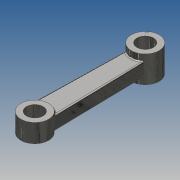
# Autodesk Inventor part: Pleuel_ra8846s
Saved by Autodesk Inventor 2021 (Build 250183000, 183)
## iProperties
Created: 2020-11-17
Part Number: Pleuel_ra8846s
Material: Stahl, hochfest, niedrig legiert
Document SubType Name: Modeling
Designer: Ricardo A
Density: 7.85031 g/cm^3
Appearance: Stahl - poliert
Description: Motor_Teil8_Pleuel
Mass: 3.359 g
Surface Area: 6.12955 cm^2
Volume: 0.427881 cm^3
Author: Sander
Revision Number: Rev00
Autodesk Inventor part; units mm, degrees
ref_plane "YZ-Ebene" through (0, 0, 0) normal (1, 0, 0) x (0, 1, 0)
ref_plane "XZ-Ebene" through (0, 0, 0) normal (0, 1, 0) x (-1, 0, 0)
ref_plane "XY-Ebene" through (0, 0, 0) normal (0, 0, 1) x (1, 0, 0)
sketch "Skizze1" plane through (0, 0, 0) normal (0, 0, 1) x (1, 0, 0)
  line L0 (-3.5, 0) -> (3.5, 0) projected
  line L1 (0, -16.8) -> (0, 16.8) projected
  line L2 (-2, 12) -> (2, 12)
  line L3 (2, 12) -> (2.5, -12)
  line L4 (2.5, -12) -> (-2.5, -12)
  line L5 (-2.5, -12) -> (-2, 12)
  point P0 (0, 0)
  dimension "d0" = 4
  dimension "d1" = 24
  dimension "d2" = 5
  constraints: 8 end point, 2 horizontal, 2 other
  measures "d0" distance of L2.start L2.end
  measures "d1" vertical distance of L2.end L3.end
  measures "d2" distance of L3.end L4.end
extrude "Extrusion1" add sketch "Skizze1" against normal mid plane 3
sketch "Skizze2" plane through (0, 0, 0) normal (0, 0, 1) x (1, 0, 0)
  line L0 (-2, 12) -> (2, 12) projected
  line L1 (-2, 12) -> (2, 12) projected
  line L2 (2, 12) -> (-2, 12) projected
  circle A0 centre (0, 12) radius 1.8
  circle A1 centre (0, 12) radius 3
  point P0 (0, 0)
  dimension "d7" = 3.6
  dimension "d8" = 6
  constraints: 2 centre point, 1 coincident, 1 midpoint
  measures "d7" diameter of A0
  measures "d8" diameter of A1
extrude "Extrusion2" add sketch "Skizze2" along normal mid plane 5.8
sketch "Skizze3" plane through (0, 0, 0) normal (0, 0, 1) x (1, 0, 0)
  line L0 (2.5, -12) -> (-2.5, -12) projected
  line L1 (-2.5, -12) -> (2.5, -12) projected
  circle A0 centre (0, -12) radius 1.8
  circle A1 centre (0, -12) radius 3
  point P0 (0, 0)
  dimension "d11" = 3.6
  dimension "d12" = 6
  constraints: 2 centre point, 1 coincident, 1 midpoint
  measures "d11" diameter of A0
  measures "d12" diameter of A1
extrude "Extrusion3" add sketch "Skizze3" along normal mid plane 4
sketch "Skizze4" plane through (0, 0, -1.5) normal (0, 0, -1) x (-1, 0, 0)
  arc A0 (1.8, -12) -> (-1.8, -12) centre (0, -12) ccw projected
  line L0 (-1.8, -12) -> (1.8, -12) projected
  point P0 (0, 0)
extrude "Extrusion4" cut sketch "Skizze4" against normal through all
sketch "Skizze5" plane through (0, 0, -1.5) normal (0, 0, -1) x (-1, 0, 0)
  arc A0 (-1.8, 12) -> (1.8, 12) centre (0, 12) ccw projected
  line L0 (1.8, 12) -> (-1.8, 12) projected
  point P0 (0, 0)
extrude "Extrusion5" cut sketch "Skizze5" against normal through all
fillet "Rundung1" radius 0.3 1 edges at (-2.255, -0.2417, -1.5)
fillet "Rundung1" radius 0.3 1 edges at (2.255, -0.2417, -1.5)
fillet "Rundung1" radius 0.3 1 edges at (-2.255, -0.2417, 1.5)
fillet "Rundung1" radius 0.3 1 edges at (2.255, -0.2417, 1.5)
fillet "Rundung2" radius 0.3 20 edges at (0, 9, 1.5) (0, -9, 1.5) (-1.959, 9.7279, 1.4126) (-2.0457, 9.8057, -0.6) (-2.0457, 9.8057, 0.6) (-1.959, 9.7279, -1.4126) (0, 9, -1.5) (1.959, 9.7279, -1.4126) (2.0457, 9.8057, -0.6) (2.0457, 9.8057, 0.6) (1.959, 9.7279, 1.4126) (2.3704, -10.1612, 1.4155) (2.4644, -10.2892, -0.6) (2.4644, -10.2892, 0.6) (2.3704, -10.1612, -1.4155) (0, -9, -1.5) (-2.3704, -10.1612, -1.4155) (-2.4644, -10.2892, -0.6) (-2.4644, -10.2892, 0.6) (-2.3704, -10.1612, 1.4155)
